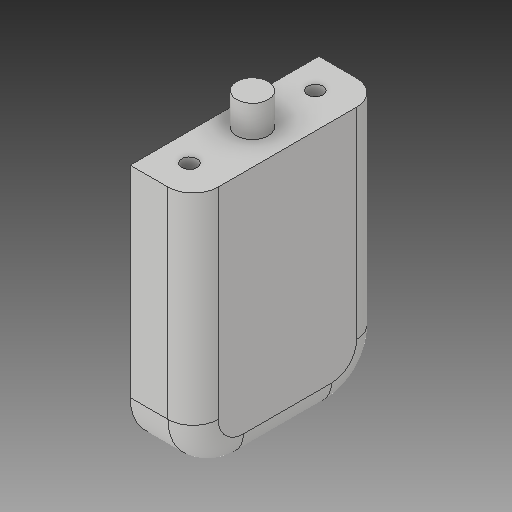
# Autodesk Inventor part: TapaPieEfector
Saved by Autodesk Inventor 2019 (Build 230136000, 136)
## iProperties
Created: 2016-12-20
Part Number: TapaPieEfector
Material: Genérico
Document SubType Name: Modeling
Designer: Mario
Density: 1 g/cm^3
Appearance: Por defecto
Author: Mario
Autodesk Inventor part; units mm, degrees
ref_plane "YZ Plane" through (0, 0, 0) normal (1, 0, 0) x (0, 1, 0)
ref_plane "XZ Plane" through (0, 0, 0) normal (0, 1, 0) x (-1, 0, 0)
ref_plane "XY Plane" through (0, 0, 0) normal (0, 0, 1) x (1, 0, 0)
sketch "Sketch1" plane through (0, 0, 0) normal (1, 0, 0) x (0, 1, 0)
  line L0 (15, 15) -> (-15, 15)
  line L1 (-15, -15) -> (15, -15)
  line L2 (15, -15) -> (15, 15)
  line L3 (15, 15) -> (-15, -15) construction
  line L4 (-15, 15) -> (15, -15) construction
  line L5 (-15, -15) -> (-25, -15)
  line L6 (-25, -15) -> (-25, 15)
  line L7 (-25, 15) -> (-15, 15)
  point P0 (0, 0)
  dimension "d0" = 30
  dimension "d1" = 30
  dimension "d13" = 10
  constraints: 16 end point, 2 horizontal, 2 midpoint, 2 perpendicular, 1 parallel
  measures "d0" distance of L1.end L1.start
  measures "d1" distance of L1.start L0.end
  measures "d13" distance of L1.start L5.end
extrude "Extrusion1" add sketch "Sketch1" along normal blind 10
sketch "Sketch2" plane through (0, 0, 0) normal (-1, 0, 0) x (0, 0, 1)
  line L0 (-13, -13) -> (-13, 13)
  line L1 (13, 13) -> (13, -13)
  line L2 (13, 13) -> (-13, 13)
  line L3 (-13, -13) -> (-13, -23)
  line L4 (-13, -23) -> (13, -23)
  line L5 (13, -23) -> (13, -13)
  point P0 (0, 0)
  dimension "d14" = 10
  constraints: 12 end point, 1 perpendicular, 1 vertical
  measures "d14" distance of L0.start L3.end
extrude "Extrusion2" cut sketch "Sketch2" against normal blind 8
sketch "Sketch3" plane through (0, 15, 15) normal (0, 1, 0) x (1, 0, 0)
  circle A0 centre (4.4342, 15) radius 2.5 projected
  point P0 (0, 15)
extrude "Extrusion3" add sketch "Sketch3" along normal blind 5
sketch "Sketch4" plane through (0, 13, -13) normal (0, -1, 0) x (1, 0, 0)
  circle A0 centre (4.4342, 23) radius 1.225 projected
  circle A1 centre (4.4342, 3) radius 1.225 projected
  point P0 (0, 13)
extrude "Extrusion4" cut sketch "Sketch4" against normal blind 2
fillet "Fillet4" radius 8 4 edges at (4, -23, 13) (4, -23, -13) (5, -25, -15) (5, -25, 15)
fillet "Fillet5" radius 4 4 edges at (10, -25, 0) (10, -22.6569, 12.6569) (10, -1, -15) (10, -22.6569, -12.6569)
sketch "Sketch11" plane through (8, 0, 0) normal (-1, 0, 0) x (0, 0, 1)
  circle A0 centre (0, -5.1293) radius 5
  circle A1 centre (0, -5.1293) radius 2.75
  point P0 (0, 0)
  dimension "d48" = 10
  constraints: 2 centre point, 1 coincident
  measures "d48" diameter of A0
extrude "Extrusion13" add sketch "Sketch11" along normal blind 8
body "Solid1"
